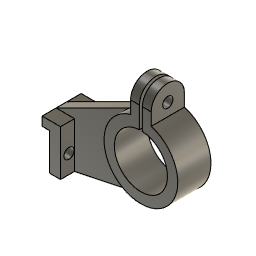
Exercise_6 v3 (Autodesk Fusion 360 design; units mm, degrees)
Autodesk Fusion 360 part; units mm, degrees
sketch "Sketch1" plane through (0, 0, 0) normal (1, 0, 0) x (0, 1, 0)
  circle A0 centre (0, 0) radius 36
  circle A1 centre (0, 0) radius 50
  line L0 (-14, 0) -> (14, 0)
  line L1 (14, 0) -> (14, 87.5)
  line L2 (14, 87.5) -> (-14, 87.5)
  line L3 (-14, 87.5) -> (-14, 0)
  line L4 (-130, -10) -> (-105, -10)
  line L5 (-105, -10) -> (-105, -72)
  line L6 (-105, -72) -> (-130, -72)
  line L7 (-130, -72) -> (-130, -10)
  line L8 (2, 87.5) -> (-2, 87.5)
  line L9 (-2, 87.5) -> (-2, 0)
  line L10 (-2, 0) -> (2, 0)
  line L11 (2, 0) -> (2, 87.5)
  line L12 (-130, -72) -> (-120, -72)
  line L13 (-120, -72) -> (-120, -22)
  line L14 (-120, -22) -> (-130, -22)
  line L15 (-130, -22) -> (-130, -72)
  line L16 (-130, -10) -> (-14, 48)
  line L17 (-105, -72) -> (0, -50)
  dimension "d1" = 72
  dimension "d2" = 100
  dimension "d3" = 87.5
  dimension "d4" = 28
  dimension "d5" = 14
  dimension "d6" = 25
  dimension "d7" = 62
  dimension "d9" = 10
  dimension "d10" = 105
  dimension "d11" = 4
  dimension "d12" = 87.5
  dimension "d16" = 10
  dimension "d17" = 50
  dimension "d18" = 87.5
  dimension "d19" = 2
  constraint coincident A0.centre A1.centre
  constraint horizontal L0
  constraint vertical L1
  constraint horizontal L2
  constraint vertical L3
  constraint horizontal L4
  constraint vertical L5
  constraint horizontal L6
  constraint vertical L7
  constraint horizontal L8
  constraint vertical L9
  constraint horizontal L10
  constraint vertical L11
  constraint coincident L2 L8.start
  constraint horizontal L12
  constraint vertical L13
  constraint horizontal L14
  constraint vertical L15
  constraint coincident A1 L16.end
  constraint coincident A1 L17.end
  measures "d1" diameter of A0
  measures "d2" diameter of A1
  measures "d3" distance of L0.end L1.end
  measures "d4" distance of L1.end L2.end
  measures "d5" distance of A0.centre L0.end
  measures "d6" distance of L4.start L4.end
  measures "d7" distance of L4.start L6.end
  measures "d9" distance of A0.centre L4
  measures "d10" distance of A0.centre L5
  measures "d11" distance of L8.start L8.end
  measures "d12" distance of L8.end L9.end
  measures "d16" distance of L6.end L12.end
  measures "d17" distance of L6.end L14.end
  measures "d18" distance of A0.centre L2
  measures "d19" distance of A0.centre L9.end
extrude "Extrude1" add sketch "Sketch1" along normal mid plane 45 contours A0 A1 L1 L3 L16 | A0 A1 L1 L11 | A0 A1 L3 L9 | A1 L1 L2 L11 | A1 L2 L3 L9 | A1 L16 makes body 1
extrude "Extrude2" add sketch "Sketch1" along normal mid plane 53 separate body contours L4 L5 L6 L7 L13 L14 makes body 2
sketch "Sketch2" plane through (0, -120, 0) normal (0, -1, 0) x (1, 0, 0)
  line L0 (-26.5, -72) -> (26.5, -72)
  line L1 (26.5, -72) -> (26.5, -22)
  line L2 (26.5, -22) -> (-26.5, -22)
  line L3 (-26.5, -22) -> (-26.5, -72)
  circle A0 centre (15, -47) radius 7
  line L4 (0, -22) -> (0, -72)
  circle A1 centre (-15, -47) radius 7
  dimension "d23" = 14
  dimension "d24" = 11.5
  dimension "d25" = 25
  constraint symmetric A0 L4 A1
  measures "d24" distance of L1 A0.centre
  measures "d25" distance of L0 A0.centre
fillet "Fillet1" radius 22.5 4 edges at (22.5, -8, 87.5) (22.5, 8, 87.5) (-22.5, -8, 87.5) (-22.5, 8, 87.5) on bodies 1
sketch "Sketch3" plane through (0, -14, 0) normal (0, -1, 0) x (1, 0, 0)
  arc A0 (22.5, 65) -> (-22.5, 65) centre (0, 65) ccw
  line L0 (-22.5, 65) -> (-22.5, 48)
  line L1 (-22.5, 48) -> (22.5, 48)
  line L2 (22.5, 48) -> (22.5, 65)
  circle A1 centre (0, 65) radius 7
  dimension "d31" = 14
  constraint concentric A0 A1
  measures "d31" diameter of A1
extrude "Extrude4" cut sketch "Sketch3" against normal up to surface (28 mm away) contours A1 bodies 1
extrude "Extrude5" cut sketch "Sketch2" against normal up to surface (15 mm away) contours A0 | A1 bodies 2
extrude "Extrude6" add sketch "Sketch1" along normal mid plane 15 contours A1 L4 L5 L16 L17 bodies 1 2
sketch "Sketch4" plane through (0, 0, 0) normal (0, 1, 0) x (1, 0, 0)
  line L0 (0, -100) -> (0, 10)
  constraint vertical L0
move_body "Move1" bodies 1 to x (0, -1, 0) y (1, 0, 0) z (0, 0, 1) at (0, 0, 0)
equation "d1 = 36 * 2 mm"
equation "d3 = 65 mm + 22.5 mm"
equation "d4 = 24 mm + 4 mm"
equation "d16 = 25 mm - 15 mm"
equation "d17 = 62 mm - 12 mm"
equation "d24 = ( ( 53 - 30 ) / 2 ) * 1 mm"
